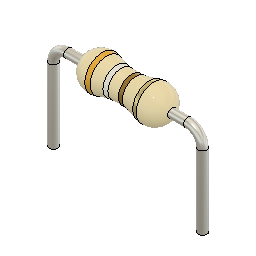
Resistor (Autodesk Fusion 360 design; units mm, degrees)
Autodesk Fusion 360 part; units mm, degrees
note: some values were not read from the file. Set by a fixed rule: which face or edge a step refers to.
sketch "Sketch1" plane through (0, 0, 0) normal (0, 0, 1) x (1, 0, 0)
  line L0 (0, 0) -> (4.5, 0)
  arc A0 (-1.4605, 1.135) -> (1.4605, 1.135) centre (0, 5.3914) ccw
  arc A1 (3.05, 0) -> (1.4605, 1.135) centre (1.85, 0) ccw
  arc A2 (-1.4605, 1.135) -> (-3.05, 0) centre (-1.85, 0) ccw
  line L1 (0, 0) -> (-4, 0)
  dimension "d1" = 2.4
  dimension "d2" = 2.4
  dimension "d3" = 9
  dimension "d5" = 3.7
  dimension "d6" = 1.85
  constraint horizontal L0.start A1.centre
  constraint horizontal L0.start A2.centre
  constraint horizontal A1.centre A1.start
  constraint horizontal A2.centre A2.end
  constraint vertical L0.start A0.centre
  constraint tangent A0 A1
  constraint coincident L0.start L1.start
  constraint horizontal L0
  constraint parallel L0 L1
  measures "d1" diameter of A1
  measures "d2" diameter of A2
  measures "d3" diameter of A0
  measures "d5" distance of A1.centre A2.centre
  measures "d6" distance of L0.start A2.centre
revolve "Revolve1" add sketch "Sketch1" angle 360 about axis through (0, 0, 0) along (1, 0, 0)
sketch "Sketch2" plane through (0, 0, 0) normal (0, 0, 1) x (1, 0, 0)
  line L0 (-1.4605, -1.135) -> (-1.4605, 1.135)
  line L1 (2.3, 0) -> (4.1, 0)
  line L2 (5.1, -1) -> (5.1, -6)
  arc A0 (5.1, -1) -> (4.1, 0) centre (4.1, -1) ccw
  line L3 (0, 0) -> (-0.5, 0) construction
  line L4 (0, 0) -> (0, 1.3)
  arc A1 (-4.1, 0) -> (-5.1, -1) centre (-4.1, -1) ccw
  line L5 (-5.1, -1) -> (-5.1, -6)
  line L6 (-2.3, 0) -> (-4.1, 0)
  dimension "d9" = 1
  dimension "d14" = 5.1
  dimension "d15" = 5
  constraint horizontal L1
  constraint tangent L1 A0
  constraint tangent L2 A0
  constraint coincident L3.start L4.start
  constraint horizontal L3
  constraint coincident L3.start L1
  constraint perpendicular L3 L4
  constraint symmetric L1.start L4 L6.start
  constraint symmetric L2.end L4 L5.end
  constraint symmetric L1.end L4 A1.start
  constraint symmetric L2.start L4 A1.end
  constraint symmetric A0 L4 A1
  constraint vertical L2
  measures "d9" radius of A0
  measures "d14" horizontal distance of L3.start L2.end
  measures "d15" distance of L2.end L2.start
pipe "Pipe1" add diameter 0.6 path "Sketch2" along L1 A0 L2
pipe "Pipe2" add diameter 0.6 path "Sketch2" along L6 A1 L5
sketch "Sketch3" plane through (0, 0, 0) normal (0, 0, 1) x (1, 0, 0)
  line L0 (-1.4605, -1.135) -> (-1.4605, 1.135)
  line L1 (-0.7605, 1.4) -> (-0.7605, -1.4)
  line L2 (-1.7605, 1.5) -> (-1.7605, -1.4)
  line L3 (-0.4605, 1.4) -> (-0.4605, -1.3)
  line L4 (0.2395, 1.4) -> (0.2395, -1.3)
  line L5 (0.5395, 1.4) -> (0.5395, -1.2)
  line L6 (1.4605, -1.135) -> (1.4605, 1.135)
  line L7 (1.7605, 1.9) -> (1.7605, -1.5)
  line L8 (-0.7605, 1.4) -> (-0.4605, 1.4)
  line L9 (0.2395, 1.4) -> (0.5395, 1.4)
  line L10 (1.4605, 1.135) -> (1.4605, 1.9)
  line L11 (1.7605, 1.9) -> (1.4605, 1.9)
  line L12 (-1.4605, 1.5) -> (-1.4605, 1.135)
  line L13 (-1.4605, 1.5) -> (-1.7605, 1.5)
  dimension "d20" = 0.3
  dimension "d21" = 0.3
  dimension "d22" = 0.3
  dimension "d23" = 0.3
  dimension "d24" = 1.7
  dimension "d25" = 0.7
  constraint parallel L0 L1
  constraint parallel L0 L2
  constraint parallel L0 L3
  constraint parallel L1 L4
  constraint parallel L3 L5
  constraint vertical L7
  constraint perpendicular L3 L8
  constraint perpendicular L5 L9
  constraint coincident L6.end L10.start
  constraint perpendicular L9 L10
  constraint perpendicular L10 L11
  constraint coincident L0.end L12.end
  constraint perpendicular L11 L12
  constraint perpendicular L2 L13
  measures "d20" distance of L0.end L2
  measures "d21" distance of L4 L5
  measures "d22" distance of L1 L3
  measures "d23" distance of L6 L7
  measures "d24" distance of L0 L4
  measures "d25" distance of L0 L1
split_face "SplitFace3" 1 faces at (-1.8655, -0.2495, -1.1737) by curves path "Sketch3" along L12 L13 L2
split_face "SplitFace5" 2 faces at (-1.2716, 1.0695, -0.107) (1.8655, 0.8917, -0.8029) by curves path "Sketch3" along L3 L8 L1
split_face "SplitFace6" 1 faces at (1.2541, 1.0684, -0.0533) by curves path "Sketch3" along L4 L9 L5
split_face "SplitFace7" 1 faces at (1.8655, 0.8917, -0.8029) by curves path "Sketch3" along L10 L11 L7
equation "d6 = d5 / 2"
equation "d14 = ( 10.2 / 2 ) * 1 mm"
